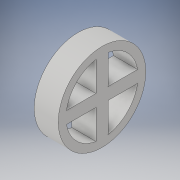
# Autodesk Inventor part: PAP
Saved by Autodesk Inventor 2018 (Build 220112000, 112)
## iProperties
Created: 2018-04-02
Part Number: PAP
Material: Generic
Document SubType Name: Modeling
Designer: Intel
Density: 1 g/cm^3
Appearance: Default
Author: Intel
Autodesk Inventor part; units mm, degrees
ref_plane "YZ Plane" through (0, 0, 0) normal (1, 0, 0) x (0, 1, 0)
ref_plane "XZ Plane" through (0, 0, 0) normal (0, 1, 0) x (-1, 0, 0)
ref_plane "XY Plane" through (0, 0, 0) normal (0, 0, 1) x (1, 0, 0)
sketch "Sketch1" plane through (0, 0, 0) normal (1, 0, 0) x (0, 1, 0)
  circle A0 centre (0, 0) radius 11.557
  arc A1 (1.3084, -9.4347) -> (9.3918, -1.5875) centre (0, 0) ccw
  arc A2 (9.3918, 1.5875) -> (1.5875, 9.3918) centre (0, 0) ccw
  arc A3 (-1.5875, 9.3918) -> (-9.3918, 1.5875) centre (0, 0) ccw
  arc A4 (-9.3918, -1.5875) -> (-1.5875, -9.3918) centre (0, 0) ccw
  line L0 (1.5875, -9.3918) -> (1.5875, -1.5875)
  line L1 (1.5875, 1.5875) -> (1.5875, 9.3918)
  line L2 (9.3918, 1.5875) -> (1.5875, 1.5875)
  line L3 (-1.5875, 1.5875) -> (-9.3918, 1.5875)
  line L4 (-1.5875, 9.3918) -> (-1.5875, 1.5875)
  line L5 (-1.5875, -1.5875) -> (-1.5875, -9.3918)
  line L6 (-9.3918, -1.5875) -> (-1.5875, -1.5875)
  line L7 (1.5875, -1.5875) -> (9.3918, -1.5875)
  dimension "d0" = 23.114
  constraints: 16 end point, 9 point on circle, 8 parallel, 5 centre point, 2 horizontal, 1 coincident
  measures "d0" diameter of A0
extrude "Extrusion1" add sketch "Sketch1" along normal blind 6.35
body "Solid1"
